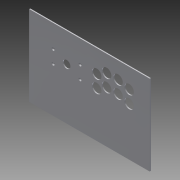
# Autodesk Inventor part: Panel_top_2
Saved by Autodesk Inventor 2013 (Build 170138000, 138)
## iProperties
Created: 2013-01-09
Part Number: Panel_top_2
Material: Aluminum
Document SubType Name: Modeling
Designer: mstine
Density: 1 g/cm^3
Author: mstine
Autodesk Inventor part; units mm, degrees
ref_plane "YZ Plane" through (0, 0, 0) normal (1, 0, 0) x (0, 1, 0)
ref_plane "XZ Plane" through (0, 0, 0) normal (0, 1, 0) x (-1, 0, 0)
ref_plane "XY Plane" through (0, 0, 0) normal (0, 0, 1) x (1, 0, 0)
sketch "Panel" plane through (0, 0, 0) normal (0, 0, 1) x (1, 0, 0)
  line L0 (-190.5, 127) -> (190.5, 127)
  line L1 (190.5, 127) -> (190.5, -127)
  line L2 (190.5, -127) -> (-190.5, -127)
  line L3 (-190.5, -127) -> (-190.5, 127)
  point P0 (0, 0)
  point P1 (-190.5, 0)
  point P2 (0, 127)
  dimension "d0" = 254
  dimension "d3" = 381
  constraints: 8 end point, 2 midpoint, 2 parallel, 1 horizontal, 1 horizontal alignment, 1 perpendicular, 1 vertical alignment
  measures "d0" distance of L2.end L0.start
  measures "d3" distance of L0.start L0.end
sketch "JoystickMount" plane through (0, 0, 0) normal (0, 0, 1) x (1, 0, 0)
  line L0 (-114.625, 55.25) -> (-114.625, 14.75) construction
  line L1 (-114.625, 14.75) -> (-29.625, 14.75) construction
  point P0 (0, 0)
  point P1 (-72.125, 35)
  point P2 (-29.625, 55.25)
  point P3 (-114.625, 35)
  point P4 (-72.125, 14.75)
  dimension "d4" = 40.5
  dimension "d6" = 85
  dimension "d19" = 35
  dimension "d45" = 72.125
  constraints: 4 end point, 3 horizontal alignment, 3 vertical alignment, 2 midpoint, 1 perpendicular, 1 vertical
  measures "d4" distance of L0.start L0.end
  measures "d6" distance of L0.end L1.end
  measures "d19" vertical distance of point (0, 0) point (-72.125, 35)
  measures "d45" horizontal distance of point (0, 0) point (-72.125, 35)
sketch "ButtonMounts" plane through (0, 0, 0) normal (0, 0, 1) x (1, 0, 0)
  line L0 (54.125, 74) -> (54.125, 35) construction
  line L1 (54.125, 35) -> (90.125, 35) construction
  point P0 (0, 0)
  point P1 (22.875, 56)
  point P2 (22.875, 17)
  point P3 (90.125, 74)
  point P4 (125.125, 65)
  point P5 (125.125, 26)
  point P6 (-72.125, 35)
  point P7 (72.125, 54.5)
  point P8 (54.125, 54.5)
  point P9 (72.125, 35)
  dimension "d7" = 39
  dimension "d9" = 39
  dimension "d10" = 39
  dimension "d11" = 39
  dimension "d12" = 31.25
  dimension "d13" = 36
  dimension "d14" = 35
  dimension "d15" = 18
  dimension "d16" = 9
  dimension "d55" = 144.25
  dimension "d56" = 72.125
  constraints: 5 vertical alignment, 4 end point, 3 horizontal alignment, 2 midpoint
  measures "d7" distance of point (22.875, 17) point (22.875, 56)
  measures "d9" distance of L0.start L0.end
  measures "d10" distance of L1.end point (90.125, 74)
  measures "d11" distance of point (125.125, 26) point (125.125, 65)
  measures "d12" horizontal distance of L0.end point (22.875, 17)
  measures "d13" distance of L0.end L1.end
  measures "d14" horizontal distance of L1.end point (125.125, 26)
  measures "d15" vertical distance of point (22.875, 17) L0.end
  measures "d16" vertical distance of point (125.125, 26) L1.end
  measures "d55" horizontal distance of point (72.125, 54.5) point (-72.125, 35)
  measures "d56" horizontal distance of point (72.125, 54.5) point (0, 0)
extrude "PanelExtrusion" add sketch "Panel" against normal blind 3.175
hole "JoystickScrews" at (-29.625, 14.75, 0) at (-29.625, 55.25, 0) at (-114.625, 55.25, 0) at (-114.625, 14.75, 0) direction (0, 0, -1) diameter 4.5 end through all countersink diameter 9.4 countersink angle 90 clearance for "Flat Head Machine Screw" size "M4" standard "Ansi Metric M Profile"
hole "JoystickShaft" at (-72.125, 35, 0) direction (0, 0, -1) diameter 24 end through all
hole "ButtonHoles" at (125.125, 26, 0) at (90.125, 35, 0) at (90.125, 74, 0) at (125.125, 65, 0) at (54.125, 74, 0) at (54.125, 35, 0) at (22.875, 56, 0) at (22.875, 17, 0) direction (0, 0, -1) diameter 30 end through all
fillet "Corners" radius 1 4 edges at (190.5, 127, -1.5875) (190.5, -127, -1.5875) (-190.5, 127, -1.5875) (-190.5, -127, -1.5875)
equation "\"d45\" = 0.5 * d55"
